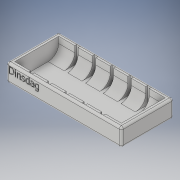
# Autodesk Inventor part: Dinsdag
Saved by Autodesk Inventor 2019 (Build 230136000, 136)
## iProperties
Created: 2020-10-20
Part Number: Dinsdag
Material: Generic
Document SubType Name: Modeling
Designer: daanswinters
Density: 1 g/cm^3
Appearance: Default
Author: daanswinters
Autodesk Inventor part; units mm, degrees
ref_plane "YZ Plane" through (0, 0, 0) normal (1, 0, 0) x (0, 1, 0)
ref_plane "XZ Plane" through (0, 0, 0) normal (0, 1, 0) x (-1, 0, 0)
ref_plane "XY Plane" through (0, 0, 0) normal (0, 0, 1) x (1, 0, 0)
sketch "Sketch1" plane through (0, 0, 0) normal (0, 0, 1) x (1, 0, 0)
  line L0 (55, -8.5) -> (-55, -8.5)
  line L1 (-55, -8.5) -> (-55, 8.5)
  line L2 (-55, 8.5) -> (55, 8.5)
  line L3 (55, 8.5) -> (55, -8.5)
  line L4 (55, -8.5) -> (-55, 8.5) construction
  line L5 (-55, -8.5) -> (55, 8.5) construction
  point P0 (0, 0)
  dimension "d0" = 110
  dimension "d1" = 17
  constraints: 12 end point, 2 midpoint, 2 parallel, 1 horizontal, 1 perpendicular
  measures "d0" distance of L1.end L2.end
  measures "d1" distance of L0.end L1.end
extrude "Extrusion1" add sketch "Sketch1" along normal blind 50
sketch "Sketch2" plane through (-55, 8.5, 0) normal (0, 1, 0) x (1, 0, 0)
  line L0 (0, 0) -> (0, -50) projected
  line L1 (110, -50) -> (0, -50)
  line L2 (0, -50) -> (0, 0)
  line L3 (0, 0) -> (110, 0)
  line L4 (110, 0) -> (110, -50)
  line L5 (110, -50) -> (0, 0) construction
  line L6 (0, -50) -> (110, 0) construction
  line L7 (106, -46) -> (106, -4)
  line L8 (4, -4) -> (4, -46)
  line L9 (56.15, -2) -> (53.85, -2)
  line L10 (53.85, -48) -> (56.15, -48)
  line L11 (56.15, -2) -> (53.85, -48) construction
  line L12 (53.85, -2) -> (56.15, -48) construction
  line L13 (73.15, -2) -> (70.85, -2)
  line L14 (70.85, -48) -> (73.15, -48)
  line L15 (73.15, -2) -> (70.85, -48) construction
  line L16 (70.85, -2) -> (73.15, -48) construction
  line L17 (0, -25) -> (110, -25) construction
  line L18 (87.85, -2) -> (90.15, -2)
  line L19 (90.15, -48) -> (87.85, -48)
  line L20 (87.85, -2) -> (90.15, -48) construction
  line L21 (90.15, -2) -> (87.85, -48) construction
  line L22 (36.85, -2) -> (39.15, -2)
  line L23 (39.15, -48) -> (36.85, -48)
  line L24 (36.85, -2) -> (39.15, -48) construction
  line L25 (39.15, -2) -> (36.85, -48) construction
  line L26 (19.85, -2) -> (22.15, -2)
  line L27 (22.15, -48) -> (19.85, -48)
  line L28 (19.85, -2) -> (22.15, -48) construction
  line L29 (22.15, -2) -> (19.85, -48) construction
  line L30 (90.15, -2) -> (90.15, -4)
  line L31 (90.15, -46) -> (90.15, -48)
  line L32 (87.85, -48) -> (87.85, -46)
  line L33 (87.85, -4) -> (87.85, -2)
  line L34 (73.15, -48) -> (73.15, -46)
  line L35 (73.15, -4) -> (73.15, -2)
  line L36 (70.85, -2) -> (70.85, -4)
  line L37 (70.85, -46) -> (70.85, -48)
  line L38 (56.15, -4) -> (56.15, -2)
  line L39 (53.85, -2) -> (53.85, -4)
  line L40 (53.85, -46) -> (53.85, -48)
  line L41 (56.15, -48) -> (56.15, -46)
  line L42 (39.15, -2) -> (39.15, -4)
  line L43 (39.15, -46) -> (39.15, -48)
  line L44 (36.85, -48) -> (36.85, -46)
  line L45 (36.85, -4) -> (36.85, -2)
  line L46 (22.15, -2) -> (22.15, -4)
  line L47 (19.85, -48) -> (19.85, -46)
  line L48 (19.85, -4) -> (19.85, -2)
  line L49 (22.15, -46) -> (22.15, -48)
  line L50 (4, -46) -> (19.95, -46)
  line L51 (22.05, -46) -> (36.95, -46)
  line L52 (39.05, -46) -> (53.95, -46)
  line L53 (56.05, -46) -> (70.95, -46)
  line L54 (73.05, -46) -> (87.95, -46)
  line L55 (90.05, -46) -> (106, -46)
  line L56 (106, -4) -> (90.05, -4)
  line L57 (87.95, -4) -> (73.05, -4)
  line L58 (70.95, -4) -> (56.05, -4)
  line L59 (53.95, -4) -> (39.05, -4)
  line L60 (36.95, -4) -> (22.05, -4)
  line L61 (19.95, -4) -> (4, -4)
  point P0 (55, 0)
  point P1 (55, -25)
  point P2 (72, -25)
  point P3 (89, -25)
  point P4 (38, -25)
  point P5 (21, -25)
  dimension "d4" = 65.556
  dimension "d5" = 110
  dimension "d7" = 2.3
  dimension "d8" = 46
  dimension "d9" = 2.3
  dimension "d10" = 46
  dimension "d11" = 0
  dimension "d12" = 2.3
  dimension "d13" = 46
  dimension "d14" = 2.3
  dimension "d15" = 46
  dimension "d16" = 2.3
  dimension "d17" = 46
  dimension "d18" = 17
  dimension "d19" = 17
  dimension "d20" = 17
  dimension "d21" = 17
  dimension "d22" = 2.862
  dimension "d23" = 2.862
  dimension "d24" = 106
  dimension "d25" = 4
  dimension "d26" = 42
  dimension "d27" = 2
  dimension "d28" = 0
  dimension "d29" = 42
  dimension "d30" = 0
  dimension "d31" = 42
  dimension "d32" = 0
  dimension "d33" = 42
  dimension "d34" = 0
  dimension "d35" = 42
  dimension "d36" = 0
  dimension "d37" = 42
  constraints: 122 end point, 73 parallel, 43 point on line, 17 perpendicular, 14 midpoint, 6 horizontal
  measures "d4" angle of L5 L0
  measures "d5" distance between parallel lines of L4 L0
  measures "d7" distance of L10.end L10.start
  measures "d8" distance of L10.start L9.end
  measures "d9" distance of L14.end L14.start
  measures "d10" distance of L14.start L13.end
  measures "d11" distance from line of L17 point (72, -25)
  measures "d12" distance of L19.start L19.end
  measures "d13" distance of L18.end L19.start
  measures "d14" distance of L23.start L23.end
  measures "d15" distance of L22.end L23.start
  measures "d16" distance of L27.start L27.end
  measures "d17" distance of L26.end L27.start
  measures "d18" distance of point (72, -25) point (55, -25)
  measures "d19" distance of point (89, -25) point (72, -25)
  measures "d20" distance of point (38, -25) point (55, -25)
  measures "d21" distance of point (21, -25) point (38, -25)
  measures "d22" angle of L0 L20
  measures "d23" angle of L0 L21
  measures "d24" distance between parallel lines of L7 L0
  measures "d25" distance between parallel lines of L8 L0
  measures "d26" distance between parallel lines of L56 L55
  measures "d27" distance between parallel lines of L56 L18
  measures "d28" distance between parallel lines of L56 L57
  measures "d29" distance between parallel lines of L56 L54
  measures "d30" distance between parallel lines of L56 L58
  measures "d31" distance between parallel lines of L56 L53
  measures "d32" distance between parallel lines of L56 L59
  measures "d33" distance between parallel lines of L56 L52
  measures "d34" distance between parallel lines of L56 L60
  measures "d35" distance between parallel lines of L56 L51
  measures "d36" distance between parallel lines of L56 L61
  measures "d37" distance between parallel lines of L56 L50
extrude "Extrusion2" cut sketch "Sketch2" against normal blind 16 contours L55 L31 L19 L32 L54 L34 L14 L37 L53 L41 L10 L40 L52 L43 L23 L44 L51 L49 L27 L47 L50 L8 L61 L48 L26 L46 L60 L45 L22 L42 L59 L39 L9 L38 L58 L36 L13 L35 L57 L33 L18 L30 L56 L7
fillet "Fillet1" radius 2 12 edges at (-55, 0, 50) (-55, 0, 0) (55, 0, 50) (55, 0, 0) (0, 8.5, 50) (-55, 8.5, 25) (0, 8.5, 0) (55, 8.5, 25) (55, -8.5, 25) (0, -8.5, 50) (-55, -8.5, 25) (0, -8.5, 0)
fillet "Fillet2" radius 10 6 edges at (-43.075, -7.5, 4) (-25.5, -7.5, 4) (-8.5, -7.5, 4) (8.5, -7.5, 4) (25.5, -7.5, 4) (43.075, -7.5, 4)
sketch "Sketch3" plane through (35.15, 8.5, 4) normal (0, 1, 0) x (1, 0, 0)
  line L0 (-70.3, -44) -> (-70.3, -42) projected
  line L1 (-51, 2) -> (-53.3, 2)
  line L2 (-34, 2) -> (-34, 0) projected
  line L3 (-36.3, -44) -> (-36.3, -42) projected
  line L4 (-19.3, -44) -> (-19.3, -42) projected
  line L5 (-2.3, -44) -> (-2.3, -42) projected
  line L6 (0, 2) -> (0, 0) projected
  line L7 (-19.8, 2) -> (-16.5, 2)
  line L8 (-16.5, 2) -> (-16.5, -44)
  line L9 (-16.5, -44) -> (-19.8, -44)
  line L10 (-19.8, -44) -> (-19.8, 2)
  line L11 (-19.8, 2) -> (-16.5, -44) construction
  line L12 (-16.5, 2) -> (-19.8, -44) construction
  line L13 (-2.8, -44) -> (0.5, -44)
  line L14 (0.5, -44) -> (0.5, 2)
  line L15 (0.5, 2) -> (-2.8, 2)
  line L16 (-2.8, 2) -> (-2.8, -44)
  line L17 (-2.8, -44) -> (0.5, 2) construction
  line L18 (0.5, -44) -> (-2.8, 2) construction
  line L19 (-36.8, -44) -> (-33.5, -44)
  line L20 (-33.5, -44) -> (-33.5, 2)
  line L21 (-33.5, 2) -> (-36.8, 2)
  line L22 (-36.8, 2) -> (-36.8, -44)
  line L23 (-36.8, -44) -> (-33.5, 2) construction
  line L24 (-33.5, -44) -> (-36.8, 2) construction
  line L25 (-51, 2) -> (-36.3, 2) projected
  line L26 (-53.8, -44) -> (-50.5, -44)
  line L27 (-50.5, -44) -> (-50.5, 2)
  line L28 (-50.5, 2) -> (-53.8, 2)
  line L29 (-53.8, 2) -> (-53.8, -44)
  line L30 (-53.8, -44) -> (-50.5, 2) construction
  line L31 (-50.5, -44) -> (-53.8, 2) construction
  line L32 (-53.3, -44) -> (-68, -44) projected
  line L33 (-70.8, 2) -> (-67.5, 2)
  line L34 (-67.5, 2) -> (-67.5, -44)
  line L35 (-67.5, -44) -> (-70.8, -44)
  line L36 (-70.8, -44) -> (-70.8, 2)
  line L37 (-70.8, 2) -> (-67.5, -44) construction
  line L38 (-67.5, 2) -> (-70.8, -44) construction
  point P0 (-35.15, 4)
  point P1 (-68, 2)
  point P2 (-17, 2)
  point P3 (-18.15, -21)
  point P4 (-1.15, -21)
  point P5 (-35.15, -21)
  point P6 (-52.15, -21)
  point P7 (-69.15, -21)
  dimension "d42" = 3.3
  dimension "d43" = 46
  dimension "d44" = 3.3
  dimension "d45" = 3.3
  dimension "d46" = 3.3
  dimension "d47" = 3.3
  dimension "d48" = 90
  dimension "d49" = 0.5
  dimension "d50" = 16.5
  dimension "d51" = 33.5
  dimension "d52" = 50.5
  dimension "d53" = 67.5
  dimension "d54" = 46
  dimension "d55" = 0
  dimension "d56" = 53.3
  constraints: 62 end point, 14 parallel, 10 midpoint, 5 horizontal, 5 perpendicular, 3 point on line
  measures "d42" distance of L8.end L9.end
  measures "d43" distance of L7.end L8.end
  measures "d44" distance of L15.end L14.end
  measures "d45" distance of L21.end L20.end
  measures "d46" distance of L28.end L27.end
  measures "d47" distance of L34.end L35.end
  measures "d48" angle of L6 L1
  measures "d49" distance between parallel lines of L6 L14
  measures "d50" distance between parallel lines of L6 L8
  measures "d51" distance between parallel lines of L6 L20
  measures "d52" distance between parallel lines of L6 L27
  measures "d53" distance between parallel lines of L6 L34
  measures "d54" distance between parallel lines of L25 L9
  measures "d55" distance between parallel lines of L15 L25
  measures "d56" distance from line of L1.end L6
extrude "Extrusion3" cut sketch "Sketch3" against normal blind 16
sketch "Sketch4" plane through (0, 0, 50) normal (0, 0, 1) x (1, 0, 0)
  line L0 (-52.9749, 6.5012) -> (53.0345, 6.5012) construction
  line L1 (53.0345, 6.5012) -> (53.0345, -6.5247) construction
  line L2 (53.0345, -6.5247) -> (-52.9749, -6.5247) construction
  line L3 (-52.9749, -6.5247) -> (-52.9749, 6.5012) construction
  spline S0 degree 2 poles (-47.5472, 3.1744) (-47.5472, 2.339) (-48.2244, 0.9944) (-48.7929, 0.6188) knots 0 0 0 1 2 2 2
  spline S1 degree 2 poles (-48.7929, 0.6188) (-49.2576, 0.3271) (-50.2116, 0.1294) (-50.9531, 0.1294) knots 0 0 0 1 2 2 2
  line L4 (-50.9531, 0.1294) -> (-52.357, 0.1294)
  line L5 (-52.357, 0.1294) -> (-52.357, 6.2294)
  line L6 (-52.357, 6.2294) -> (-50.968, 6.2294)
  spline S2 degree 2 poles (-50.968, 6.2294) (-50.1078, 6.2294) (-49.1291, 5.9723) (-48.783, 5.7449) knots 0 0 0 1 2 2 2
  spline S3 degree 2 poles (-48.783, 5.7449) (-48.1948, 5.3544) (-47.5472, 4.0642) (-47.5472, 3.1744) knots 0 0 0 1 2 2 2
  spline S4 degree 2 poles (-48.3925, 3.1843) (-48.3925, 3.8863) (-48.8572, 4.8799) (-49.3169, 5.1616) knots 0 0 0 1 2 2 2
  spline S5 degree 2 poles (-49.3169, 5.1616) (-49.6432, 5.3544) (-50.3797, 5.5274) (-50.9284, 5.5274) knots 0 0 0 1 2 2 2
  line L7 (-50.9284, 5.5274) -> (-51.5463, 5.5274)
  line L8 (-51.5463, 5.5274) -> (-51.5463, 0.8313)
  line L9 (-51.5463, 0.8313) -> (-50.9284, 0.8313)
  spline S6 degree 2 poles (-50.9284, 0.8313) (-50.3896, 0.8313) (-49.574, 1.0043) (-49.2428, 1.2367) knots 0 0 0 1 2 2 2
  spline S7 degree 2 poles (-49.2428, 1.2367) (-48.8176, 1.5234) (-48.3925, 2.4725) (-48.3925, 3.1843) knots 0 0 0 1 2 2 2
  line L10 (-45.9406, 0.1294) -> (-46.7118, 0.1294)
  line L11 (-46.7118, 0.1294) -> (-46.7118, 4.7068)
  line L12 (-46.7118, 4.7068) -> (-45.9406, 4.7068)
  line L13 (-45.9406, 4.7068) -> (-45.9406, 0.1294)
  line L14 (-45.8863, 5.4681) -> (-46.7612, 5.4681)
  line L15 (-46.7612, 5.4681) -> (-46.7612, 6.2689)
  line L16 (-46.7612, 6.2689) -> (-45.8863, 6.2689)
  line L17 (-45.8863, 6.2689) -> (-45.8863, 5.4681)
  line L18 (-41.2149, 0.1294) -> (-41.986, 0.1294)
  line L19 (-41.986, 0.1294) -> (-41.986, 2.7394)
  spline S8 degree 2 poles (-41.986, 2.7394) (-41.986, 3.0558) (-42.0453, 3.5995) (-42.1343, 3.7627) knots 0 0 0 1 2 2 2
  spline S9 degree 2 poles (-42.1343, 3.7627) (-42.2282, 3.9357) (-42.5644, 4.1038) (-42.8511, 4.1038) knots 0 0 0 1 2 2 2
  spline S10 degree 2 poles (-42.8511, 4.1038) (-43.1378, 4.1038) (-43.7458, 3.7973) (-44.0375, 3.5501) knots 0 0 0 1 2 2 2
  line L20 (-44.0375, 3.5501) -> (-44.0375, 0.1294)
  line L21 (-44.0375, 0.1294) -> (-44.8086, 0.1294)
  line L22 (-44.8086, 0.1294) -> (-44.8086, 4.7068)
  line L23 (-44.8086, 4.7068) -> (-44.0375, 4.7068)
  line L24 (-44.0375, 4.7068) -> (-44.0375, 4.1977)
  spline S11 degree 2 poles (-44.0375, 4.1977) (-43.6915, 4.5091) (-43.0241, 4.8354) (-42.6484, 4.8354) knots 0 0 0 1 2 2 2
  spline S12 degree 2 poles (-42.6484, 4.8354) (-41.9761, 4.8354) (-41.2149, 3.9456) (-41.2149, 3.1003) knots 0 0 0 1 2 2 2
  line L25 (-41.2149, 3.1003) -> (-41.2149, 0.1294)
  spline S13 degree 2 poles (-38.8965, 0.0206) (-39.3562, 0.0206) (-40.1521, 0.2678) (-40.4141, 0.4062) knots 0 0 0 1 2 2 2
  line L26 (-40.4141, 0.4062) -> (-40.4141, 1.2713)
  line L27 (-40.4141, 1.2713) -> (-40.3745, 1.2713)
  spline S14 degree 2 poles (-40.3745, 1.2713) (-40.2757, 1.1922) (-40.0087, 1.0043) (-39.7863, 0.9005) knots 0 0 0 1 2 2 2
  spline S15 degree 2 poles (-39.7863, 0.9005) (-39.5935, 0.8066) (-39.1189, 0.6682) (-38.8668, 0.6682) knots 0 0 0 1 2 2 2
  spline S16 degree 2 poles (-38.8668, 0.6682) (-38.6839, 0.6682) (-38.2637, 0.7522) (-38.1649, 0.8214) knots 0 0 0 1 2 2 2
  spline S17 degree 2 poles (-38.1649, 0.8214) (-38.0215, 0.9153) (-37.893, 1.1279) (-37.893, 1.3454) knots 0 0 0 1 2 2 2
  spline S18 degree 2 poles (-37.893, 1.3454) (-37.893, 1.6173) (-38.1896, 1.8991) (-38.5702, 1.993) knots 0 0 0 1 2 2 2
  spline S19 degree 2 poles (-38.5702, 1.993) (-38.7185, 2.0276) (-39.1931, 2.1265) (-39.3958, 2.1808) knots 0 0 0 1 2 2 2
  spline S20 degree 2 poles (-39.3958, 2.1808) (-39.9197, 2.3341) (-40.3943, 2.9668) (-40.3943, 3.4166) knots 0 0 0 1 2 2 2
  spline S21 degree 2 poles (-40.3943, 3.4166) (-40.3943, 4.0395) (-39.46, 4.8156) (-38.6889, 4.8156) knots 0 0 0 1 2 2 2
  spline S22 degree 2 poles (-38.6889, 4.8156) (-38.3082, 4.8156) (-37.5371, 4.6277) (-37.2751, 4.4844) knots 0 0 0 1 2 2 2
  line L28 (-37.2751, 4.4844) -> (-37.2751, 3.6589)
  line L29 (-37.2751, 3.6589) -> (-37.3146, 3.6589)
  spline S23 degree 2 poles (-37.3146, 3.6589) (-37.6112, 3.8961) (-38.3329, 4.168) (-38.7037, 4.168) knots 0 0 0 1 2 2 2
  spline S24 degree 2 poles (-38.7037, 4.168) (-39.0843, 4.168) (-39.6083, 3.8467) (-39.6083, 3.5254) knots 0 0 0 1 2 2 2
  spline S25 degree 2 poles (-39.6083, 3.5254) (-39.6083, 3.2337) (-39.2969, 2.952) (-38.9509, 2.863) knots 0 0 0 1 2 2 2
  spline S26 degree 2 poles (-38.9509, 2.863) (-38.7828, 2.8185) (-38.3577, 2.7295) (-38.1253, 2.6752) knots 0 0 0 1 2 2 2
  spline S27 degree 2 poles (-38.1253, 2.6752) (-37.6211, 2.5466) (-37.107, 1.9584) (-37.107, 1.4492) knots 0 0 0 1 2 2 2
  spline S28 degree 2 poles (-37.107, 1.4492) (-37.107, 1.1526) (-37.3394, 0.6286) (-37.5667, 0.4359) knots 0 0 0 1 2 2 2
  spline S29 degree 2 poles (-37.5667, 0.4359) (-37.809, 0.2332) (-38.4269, 0.0206) (-38.8965, 0.0206) knots 0 0 0 1 2 2 2
  line L30 (-32.8706, 0.1294) -> (-33.6418, 0.1294)
  line L31 (-33.6418, 0.1294) -> (-33.6418, 0.594)
  spline S30 degree 2 poles (-33.6418, 0.594) (-33.8197, 0.4457) (-34.0817, 0.248) (-34.2597, 0.164) knots 0 0 0 1 2 2 2
  spline S31 degree 2 poles (-34.2597, 0.164) (-34.4228, 0.0849) (-34.7738, 0.0008) (-35.0061, 0.0008) knots 0 0 0 1 2 2 2
  spline S32 degree 2 poles (-35.0061, 0.0008) (-35.3818, 0.0008) (-36.0146, 0.3123) (-36.237, 0.6138) knots 0 0 0 1 2 2 2
  spline S33 degree 2 poles (-36.237, 0.6138) (-36.4594, 0.9153) (-36.7066, 1.8051) (-36.7066, 2.3835) knots 0 0 0 1 2 2 2
  spline S34 degree 2 poles (-36.7066, 2.3835) (-36.7066, 2.9866) (-36.3952, 3.8665) (-36.1233, 4.1977) knots 0 0 0 1 2 2 2
  spline S35 degree 2 poles (-36.1233, 4.1977) (-35.8712, 4.4943) (-35.1643, 4.8354) (-34.7738, 4.8354) knots 0 0 0 1 2 2 2
  spline S36 degree 2 poles (-34.7738, 4.8354) (-34.4327, 4.8354) (-33.9235, 4.6821) (-33.6418, 4.5239) knots 0 0 0 1 2 2 2
  line L32 (-33.6418, 4.5239) -> (-33.6418, 6.5012)
  line L33 (-33.6418, 6.5012) -> (-32.8706, 6.5012)
  line L34 (-32.8706, 6.5012) -> (-32.8706, 0.1294)
  line L35 (-33.6418, 1.2416) -> (-33.6418, 3.8863)
  spline S37 degree 2 poles (-33.6418, 3.8863) (-33.9285, 4.0247) (-34.3833, 4.1285) (-34.6453, 4.1285) knots 0 0 0 1 2 2 2
  spline S38 degree 2 poles (-34.6453, 4.1285) (-35.2385, 4.1285) (-35.9107, 3.2387) (-35.9107, 2.3983) knots 0 0 0 1 2 2 2
  spline S39 degree 2 poles (-35.9107, 2.3983) (-35.9107, 1.5876) (-35.3966, 0.7324) (-34.8282, 0.7324) knots 0 0 0 1 2 2 2
  spline S40 degree 2 poles (-34.8282, 0.7324) (-34.5266, 0.7324) (-33.9137, 1.0093) (-33.6418, 1.2416) knots 0 0 0 1 2 2 2
  spline S41 degree 2 poles (-29.2027, 0.6138) (-29.2966, 0.5446) (-29.613, 0.2974) (-29.7613, 0.2233) knots 0 0 0 1 2 2 2
  spline S42 degree 2 poles (-29.7613, 0.2233) (-29.964, 0.1145) (-30.3446, 0.0008) (-30.6906, 0.0008) knots 0 0 0 1 2 2 2
  spline S43 degree 2 poles (-30.6906, 0.0008) (-30.9724, 0.0008) (-31.4816, 0.2134) (-31.6744, 0.4062) knots 0 0 0 1 2 2 2
  spline S44 degree 2 poles (-31.6744, 0.4062) (-31.8573, 0.594) (-32.0797, 1.1477) (-32.0797, 1.4542) knots 0 0 0 1 2 2 2
  spline S45 degree 2 poles (-32.0797, 1.4542) (-32.0797, 1.9287) (-31.6793, 2.601) (-31.2443, 2.7938) knots 0 0 0 1 2 2 2
  spline S46 degree 2 poles (-31.2443, 2.7938) (-30.8587, 2.9718) (-29.8107, 3.1052) (-29.2027, 3.1398) knots 0 0 0 1 2 2 2
  line L36 (-29.2027, 3.1398) -> (-29.2027, 3.2881)
  spline S47 degree 2 poles (-29.2027, 3.2881) (-29.2027, 3.5551) (-29.3658, 3.8863) (-29.5141, 3.9802) knots 0 0 0 1 2 2 2
  spline S48 degree 2 poles (-29.5141, 3.9802) (-29.6624, 4.0741) (-30.0876, 4.1334) (-30.315, 4.1334) knots 0 0 0 1 2 2 2
  spline S49 degree 2 poles (-30.315, 4.1334) (-30.5819, 4.1334) (-31.3036, 3.9752) (-31.6645, 3.822) knots 0 0 0 1 2 2 2
  line L37 (-31.6645, 3.822) -> (-31.709, 3.822)
  line L38 (-31.709, 3.822) -> (-31.709, 4.608)
  spline S50 degree 2 poles (-31.709, 4.608) (-31.4964, 4.6673) (-30.7005, 4.8156) (-30.31, 4.8156) knots 0 0 0 1 2 2 2
  spline S51 degree 2 poles (-30.31, 4.8156) (-29.8355, 4.8156) (-29.1879, 4.6673) (-28.9308, 4.4745) knots 0 0 0 1 2 2 2
  spline S52 degree 2 poles (-28.9308, 4.4745) (-28.6787, 4.2867) (-28.4316, 3.6885) (-28.4316, 3.2585) knots 0 0 0 1 2 2 2
  line L39 (-28.4316, 3.2585) -> (-28.4316, 0.1294)
  line L40 (-28.4316, 0.1294) -> (-29.2027, 0.1294)
  line L41 (-29.2027, 0.1294) -> (-29.2027, 0.6138)
  line L42 (-29.2027, 1.2564) -> (-29.2027, 2.5269)
  spline S53 degree 2 poles (-29.2027, 2.5269) (-29.4795, 2.5021) (-30.315, 2.4181) (-30.577, 2.339) knots 0 0 0 1 2 2 2
  spline S54 degree 2 poles (-30.577, 2.339) (-30.8834, 2.2451) (-31.2838, 1.8546) (-31.2838, 1.5085) knots 0 0 0 1 2 2 2
  spline S55 degree 2 poles (-31.2838, 1.5085) (-31.2838, 1.1131) (-30.8389, 0.7127) (-30.4138, 0.7127) knots 0 0 0 1 2 2 2
  spline S56 degree 2 poles (-30.4138, 0.7127) (-30.053, 0.7127) (-29.4598, 1.0241) (-29.2027, 1.2564) knots 0 0 0 1 2 2 2
  spline S57 degree 2 poles (-27.1859, -0.6022) (-27.1068, -0.6368) (-26.8052, -0.7456) (-26.6124, -0.7901) knots 0 0 0 1 2 2 2
  spline S58 degree 2 poles (-26.6124, -0.7901) (-26.3999, -0.8445) (-26.039, -0.9087) (-25.8265, -0.9087) knots 0 0 0 1 2 2 2
  spline S59 degree 2 poles (-25.8265, -0.9087) (-25.4706, -0.9087) (-24.9762, -0.7209) (-24.8378, -0.5528) knots 0 0 0 1 2 2 2
  spline S60 degree 2 poles (-24.8378, -0.5528) (-24.7043, -0.3847) (-24.6005, 0.0552) (-24.6005, 0.337) knots 0 0 0 1 2 2 2
  line L43 (-24.6005, 0.337) -> (-24.6005, 0.7374)
  spline S61 degree 2 poles (-24.6005, 0.7374) (-24.912, 0.4655) (-25.5101, 0.2085) (-25.9599, 0.2085) knots 0 0 0 1 2 2 2
  spline S62 degree 2 poles (-25.9599, 0.2085) (-26.741, 0.2085) (-27.6654, 1.3701) (-27.6654, 2.4626) knots 0 0 0 1 2 2 2
  spline S63 degree 2 poles (-27.6654, 2.4626) (-27.6654, 3.0311) (-27.3441, 3.911) (-27.0771, 4.2224) knots 0 0 0 1 2 2 2
  spline S64 degree 2 poles (-27.0771, 4.2224) (-26.8201, 4.5141) (-26.1132, 4.8354) (-25.7375, 4.8354) knots 0 0 0 1 2 2 2
  spline S65 degree 2 poles (-25.7375, 4.8354) (-25.3816, 4.8354) (-24.8625, 4.6673) (-24.6005, 4.5141) knots 0 0 0 1 2 2 2
  line L44 (-24.6005, 4.5141) -> (-24.556, 4.7068)
  line L45 (-24.556, 4.7068) -> (-23.8294, 4.7068)
  line L46 (-23.8294, 4.7068) -> (-23.8294, 0.6534)
  spline S66 degree 2 poles (-23.8294, 0.6534) (-23.8294, -0.5133) (-24.8428, -1.6008) (-25.8858, -1.6008) knots 0 0 0 1 2 2 2
  spline S67 degree 2 poles (-25.8858, -1.6008) (-26.2219, -1.6008) (-26.9239, -1.492) (-27.2254, -1.403) knots 0 0 0 1 2 2 2
  line L47 (-27.2254, -1.403) -> (-27.2254, -0.6022)
  line L48 (-27.2254, -0.6022) -> (-27.1859, -0.6022)
  line L49 (-24.6005, 1.3701) -> (-24.6005, 3.8863)
  spline S68 degree 2 poles (-24.6005, 3.8863) (-24.8872, 4.0247) (-25.3717, 4.1433) (-25.6139, 4.1433) knots 0 0 0 1 2 2 2
  spline S69 degree 2 poles (-25.6139, 4.1433) (-26.1972, 4.1433) (-26.8695, 3.2832) (-26.8695, 2.4774) knots 0 0 0 1 2 2 2
  spline S70 degree 2 poles (-26.8695, 2.4774) (-26.8695, 1.7162) (-26.3603, 0.9203) (-25.7869, 0.9203) knots 0 0 0 1 2 2 2
  spline S71 degree 2 poles (-25.7869, 0.9203) (-25.4854, 0.9203) (-24.8526, 1.1576) (-24.6005, 1.3701) knots 0 0 0 1 2 2 2
  point P0 (0, 0)
  constraints: 2 other
extrude "Extrusion4" cut sketch "Sketch4" against normal blind 0.5
fillet "Fillet3" radius 10 6 edges at (-43.325, -7.5, 46) (-25.5, -7.5, 46) (-8.5, -7.5, 46) (8.5, -7.5, 46) (25.5, -7.5, 46) (43.325, -7.5, 46)
body "Solid1"
